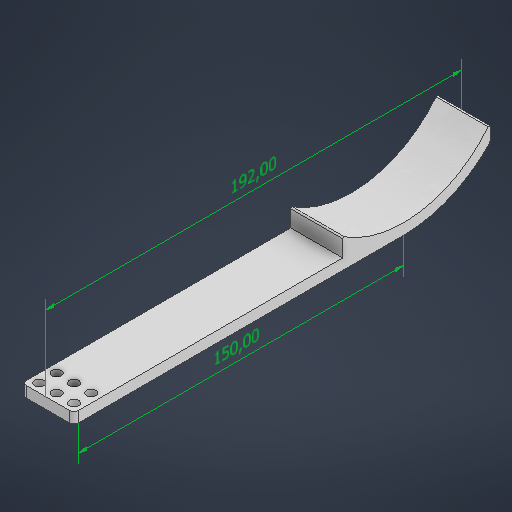
# Autodesk Inventor part: Launcher_Arm_V1
Saved by Autodesk Inventor 2026.1 (Build 301233020, 233B)
## iProperties
Created: 2025-11-02
Part Number: Launcher_Arm_V1
Material: Generic
Document SubType Name: Modeling
Designer: Asus
Density: 1 g/cm^3
Appearance: Default
Author: Asus
Autodesk Inventor part; units mm, degrees
ref_plane "YZ Plane" through (0, 0, 0) normal (1, 0, 0) x (0, 1, 0)
ref_plane "XZ Plane" through (0, 0, 0) normal (0, 1, 0) x (-1, 0, 0)
ref_plane "XY Plane" through (0, 0, 0) normal (0, 0, 1) x (1, 0, 0)
sketch "Sketch1" plane through (0, 0, 0) normal (0, 1, 0) x (-1, 0, 0)
  line L0 (-10, 96) -> (10, 96)
  line L1 (12, 94) -> (12, -96)
  line L2 (12, -96) -> (-12, -96)
  line L3 (-12, -96) -> (-12, 94)
  line L4 (-12, 96) -> (12, -96) construction
  line L5 (12, 96) -> (-12, -96) construction
  arc A0 (12, 94) -> (10, 96) centre (10, 94) ccw
  arc A1 (-10, 96) -> (-12, 94) centre (-10, 94) ccw
  circle A2 centre (8, 92) radius 2.2
  circle A3 centre (0, 92) radius 2.2
  circle A4 centre (-8, 92) radius 2.2
  circle A5 centre (8, 84) radius 2.2
  circle A6 centre (0, 84) radius 2.2
  circle A7 centre (-8, 84) radius 2.2
  point P0 (0, 0)
  dimension "d0" = 24
  dimension "d1" = 192
  dimension "d2" = 2
  dimension "d3" = 4.4
  dimension "d4" = 4
  dimension "d5" = 4
  dimension "d8" = 8
  dimension "d11" = 8
  constraints: 12 end point, 8 centre point, 4 point on circle, 4 point on line, 4 tangent, 2 horizontal, 2 midpoint, 2 parallel, 1 equal radius, 1 perpendicular, 1 vertical, 10 other
  measures "d0" distance of L1.end L2.end
  measures "d1" distance of L5.start L1.end
  measures "d2" radius of A0
  measures "d3" diameter of A2
  measures "d4" distance from line of L1 A2.centre
  measures "d5" distance from line of L0 A2.centre
  measures "d8" distance of A2.centre A3.centre
  measures "d11" distance of A2.centre A5.centre
extrude "Extrusion1" add sketch "Sketch1" along normal blind 5
sketch "Sketch2" plane through (12, 0, 94) normal (1, 0, 0) x (0, 0, -1)
  arc A0 (150, 5) -> (189.1089, 23.8473) centre (150, 55) ccw
  line L0 (0, 5) -> (190, 5) projected
  line L1 (190, 5) -> (190, 23.5357)
  arc A1 (190, 23.5357) -> (189.1089, 23.8473) centre (189.5, 23.5357) ccw
  point P0 (94, 0)
  point P1 (190, 25)
  dimension "d16" = 100
  dimension "d17" = 40
  dimension "d18" = 0.5
  constraints: 5 point on circle, 3 tangent, 2 centre point, 2 end point, 2 point on line, 1 vertical
  measures "d16" diameter of A0
  measures "d17" distance from line of L1 A0.centre
  measures "d18" radius of A1
extrude "Extrusion2" add sketch "Sketch2" against normal blind 24
sketch "Sketch3" plane through (12, 0, 94) normal (1, 0, 0) x (0, 0, -1)
  line L0 (0, 0) -> (190, 0) projected
  arc A0 (150, 5) -> (189.1089, 23.8473) centre (150, 55) ccw projected
  line L1 (0, 5) -> (150, 5) projected
  arc A1 (150, 0) -> (189.8624, 17.1055) centre (150, 55) ccw
  line L2 (190, 0) -> (190, 23.5357) projected
  line L3 (190, 17.2508) -> (190, 0)
  line L4 (190, 0) -> (150, 0)
  arc A2 (189.8624, 17.1055) -> (190, 17.45) centre (189.5, 17.45) ccw
  point P0 (150, 0)
  dimension "d27" = 1
  dimension "d28" = 17.2508
  constraints: 4 end point, 4 point on circle, 3 tangent, 2 centre point, 2 point on line, 1 coincident, 1 vertical
  measures "d27" diameter of A2
  measures "d28" distance of L0.end L3.start
extrude "Extrusion3" cut sketch "Sketch3" against normal blind 24
sketch "Sketch4" plane through (12, 0, 94) normal (1, 0, 0) x (0, 0, -1)
  arc A0 (122.7723, 13.0637) -> (150, 5) centre (150, 55) ccw
  line L0 (0, 5) -> (150, 5) projected
  line L1 (190, 17.45) -> (190, 23.5357) projected
  line L2 (122, 5) -> (122, 12.6444)
  arc A1 (122.7723, 13.0637) -> (122, 12.6444) centre (122.5, 12.6444) ccw
  point P0 (94, 0)
  point P1 (122, 13.5754)
  dimension "d31" = 0.5
  constraints: 5 point on circle, 3 end point, 3 tangent, 2 centre point, 2 point on line, 1 perpendicular
  measures "d31" radius of A1
extrude "Extrusion4" add sketch "Sketch4" against normal blind 24
body "Solid1"
